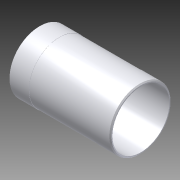
# Autodesk Inventor part: 13_0204_039
Saved by Autodesk Inventor 2012 SP1 (Build 160190100, 190)
## iProperties
Created: 2013-04-04
Part Number: 13_0204_039
Material: Default
Document SubType Name: Modeling
Designer: vogel
Density: 1 g/cm^3
Author: vogel
Autodesk Inventor part; units mm, degrees
ref_plane "YZ Plane" through (0, 0, 0) normal (1, 0, 0) x (0, 1, 0)
ref_plane "XZ Plane" through (0, 0, 0) normal (0, 1, 0) x (-1, 0, 0)
ref_plane "XY Plane" through (0, 0, 0) normal (0, 0, 1) x (1, 0, 0)
sketch "Skizze1" plane through (0, 0, 0) normal (0, 0, 1) x (1, 0, 0)
  line L0 (-60, 0) -> (10, 0) projected
  line L1 (0, -3) -> (0, 18) projected
  line L2 (0, 14) -> (-50, 14)
  line L3 (-50, 14) -> (-50, 15)
  line L4 (-50, 15) -> (-40, 15)
  line L5 (-40, 15) -> (-40, 14.9)
  line L6 (-40, 14.9) -> (-10, 14.9)
  line L7 (-10, 14.9) -> (-10, 15)
  line L8 (-10, 15) -> (0, 15)
  line L9 (0, 14) -> (0, 15)
  point P0 (0, 0)
  dimension "d1" = 28
  dimension "d2" = 30
  dimension "d4" = 50
  dimension "d5" = 10
  dimension "d6" = 10
  dimension "d11" = 0.1
  constraints: 16 end point, 4 parallel, 3 perpendicular, 2 collinear, 2 point on line
  measures "d1" diameter of L2 L0
  measures "d2" diameter of L8 L0
  measures "d4" distance of L2.start L2.end
  measures "d5" distance of L7.end L8.end
  measures "d6" distance of L3.end L4.end
  measures "d11" distance between parallel lines of L6 L8
revolve "Umdrehung1" add sketch "Skizze1" angle 360 about axis through (-10, 0, 0) along (1, 0, 0)
chamfer "Fase1" distance 0.5 angle 45 2 edges at (0, -15, 0) (-50, -15, 0)
